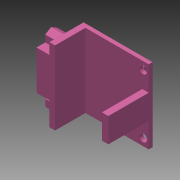
# Autodesk Inventor part: RS 232 Board
Saved by Autodesk Inventor 2015 SP1 (Build 190203100, 203)
## iProperties
Created: 2015-03-22
Part Number: RS 232 Board
Material: Generic
Document SubType Name: Modeling
Designer: steele
Density: 1 g/cm^3
Appearance: Pink
Author: steele
Autodesk Inventor part; units mm, degrees
ref_plane "YZ Plane" through (0, 0, 0) normal (1, 0, 0) x (0, 1, 0)
ref_plane "XZ Plane" through (0, 0, 0) normal (0, 1, 0) x (-1, 0, 0)
ref_plane "XY Plane" through (0, 0, 0) normal (0, 0, 1) x (1, 0, 0)
sketch "Sketch1" plane through (0, 0, 0) normal (0, 1, 0) x (-1, 0, 0)
  line L0 (14.5, -15.5) -> (-14.5, -15.5)
  line L1 (-14.5, -15.5) -> (-14.5, 15.5)
  line L2 (-14.5, 15.5) -> (14.5, 15.5)
  line L3 (14.5, 15.5) -> (14.5, -15.5)
  line L4 (14.5, -15.5) -> (-14.5, 15.5) construction
  line L5 (-14.5, -15.5) -> (14.5, 15.5) construction
  point P0 (0, 0)
  dimension "d0" = 29
  dimension "d1" = 31
  constraints: 12 end point, 2 midpoint, 2 parallel, 1 horizontal, 1 perpendicular
  measures "d0" distance of L0.start L0.end
  measures "d1" distance of L0.end L1.end
extrude "Extrusion1" add sketch "Sketch1" along normal blind 1.6
sketch "Sketch2" plane through (0, 0, 0) normal (0, -1, 0) x (1, 0, 0)
  line L0 (-14.5, 15.5) -> (-12.1, 15.5)
  line L1 (-12.1, 15.5) -> (-12.1, -15.5)
  line L2 (-12.1, -15.5) -> (-14.5, -15.5)
  line L3 (-14.5, -15.5) -> (-14.5, 15.5)
  point P0 (0, 0)
  dimension "d4" = 2.4
  constraints: 8 end point, 2 parallel, 1 horizontal, 1 perpendicular
  measures "d4" distance between parallel lines of L3 L1
extrude "Extrusion2" add sketch "Sketch2" along normal blind 12.8
sketch "Sketch3" plane through (0, 0, 0) normal (0, -1, 0) x (1, 0, 0)
  line L0 (-14.5, 15.5) -> (14.5, 15.5) construction
  line L1 (12.125, 15.5) -> (12.125, -15.5904) construction
  line L2 (14.5, -15.5) -> (14.5, 15.5) construction
  line L3 (12.125, 12.375) -> (14.5, 12.375) construction
  line L4 (12.125, -12.375) -> (14.5, -12.375) construction
  line L5 (-12.1, -15.5) -> (14.5, -15.5) construction
  circle A0 centre (12.125, 12.375) radius 1.625
  circle A1 centre (12.125, -12.375) radius 1.625
  point P0 (0, 0)
  dimension "d7" = 2.375
  dimension "d8" = 3.125
  dimension "d9" = 3.125
  dimension "d10" = 3.25
  constraints: 6 end point, 5 point on line, 2 centre point, 2 coincident, 1 equal radius, 1 parallel, 1 perpendicular, 1 vertical
  measures "d7" distance between parallel lines of L1 L2
  measures "d8" distance between parallel lines of L0 L3
  measures "d9" distance between parallel lines of L5 L4
  measures "d10" diameter of A0
extrude "Extrusion3" cut sketch "Sketch3" against normal through all
sketch "Sketch4" plane through (-14.5, 1.6, -15.5) normal (-1, 0, 0) x (0, 0, 1)
  line L0 (30.9539, -7.65) -> (0, -7.65) construction
  line L1 (0, -14.4) -> (0, 0) construction
  line L2 (0, 0) -> (31, 0) construction
  line L3 (24.3332, -7.65) -> (25.7766, -5.15)
  line L4 (25.7766, -5.15) -> (28.6634, -5.15)
  line L5 (28.6634, -5.15) -> (30.1068, -7.65)
  line L6 (30.1068, -7.65) -> (28.6634, -10.15)
  line L7 (28.6634, -10.15) -> (25.7766, -10.15)
  line L8 (25.7766, -10.15) -> (24.3332, -7.65)
  line L9 (2.3366, -10.15) -> (0.8932, -7.65)
  line L10 (0.8932, -7.65) -> (2.3366, -5.15)
  line L11 (2.3366, -5.15) -> (5.2234, -5.15)
  line L12 (5.2234, -5.15) -> (6.6668, -7.65)
  line L13 (6.6668, -7.65) -> (5.2234, -10.15)
  line L14 (5.2234, -10.15) -> (2.3366, -10.15)
  line L15 (31, 0) -> (31, -14.4) projected
  point P0 (15.5, -1.6)
  point P1 (27.22, -7.65)
  point P2 (3.78, -7.65)
  dimension "d13" = 7.65
  dimension "d14" = 5
  dimension "d15" = 3.78
  dimension "d16" = 3.78
  constraints: 26 end point, 3 parallel, 3 point on line, 1 horizontal, 26 other
  measures "d13" distance between parallel lines of L0 L2
  measures "d14" distance between parallel lines of L4 L7
  measures "d15" distance from line of L15 point (27.22, -7.65)
  measures "d16" distance from line of L1 point (3.78, -7.65)
extrude "Extrusion4" add sketch "Sketch4" along normal blind 6
sketch "Sketch5" plane through (-14.5, 1.6, -15.5) normal (-1, 0, 0) x (0, 0, 1)
  line L0 (0, 0) -> (31, 0) construction
  line L1 (15.5, 0) -> (15.5, -14.4) construction
  line L2 (31, -14.4) -> (0, -14.4) construction
  line L3 (23.75, -3.8) -> (7.25, -3.8)
  line L4 (7.25, -3.8) -> (7.25, -11.8)
  line L5 (7.25, -11.8) -> (23.75, -11.8)
  line L6 (23.75, -11.8) -> (23.75, -3.8)
  line L7 (23.75, -3.8) -> (7.25, -11.8) construction
  line L8 (7.25, -3.8) -> (23.75, -11.8) construction
  point P0 (15.5, -1.6)
  point P1 (15.5, -7.8)
  dimension "d19" = 3.8
  dimension "d20" = 8
  dimension "d21" = 16.5
  constraints: 14 end point, 4 midpoint, 2 parallel, 1 horizontal, 1 perpendicular, 1 point on line
  measures "d19" distance between parallel lines of L3 L0
  measures "d20" distance of L5.end L3.start
  measures "d21" distance of L4.end L5.end
extrude "Extrusion5" add sketch "Sketch5" along normal blind 8
sketch "Sketch6" plane through (0, 1.6, 0) normal (0, 1, 0) x (1, 0, 0)
  line L0 (9.5, -10.5) -> (9.5, 10.5)
  line L1 (9.5, 10.5) -> (-9.5, 10.5)
  line L2 (-9.5, 10.5) -> (-9.5, -10.5)
  line L3 (-9.5, -10.5) -> (9.5, -10.5)
  line L4 (9.5, -10.5) -> (-9.5, 10.5) construction
  line L5 (9.5, 10.5) -> (-9.5, -10.5) construction
  line L6 (14.5, -15.5) -> (14.5, 15.5) projected
  line L7 (-14.5, -15.5) -> (14.5, -15.5) projected
  point P0 (0, 0)
  dimension "d24" = 5
  dimension "d25" = 5
  constraints: 12 end point, 2 midpoint, 2 parallel, 1 perpendicular, 1 vertical
  measures "d24" distance between parallel lines of L0 L6
  measures "d25" distance between parallel lines of L3 L7
extrude "Extrusion6" add sketch "Sketch6" along normal blind 3
sketch "Sketch7" plane through (0, 0, 0) normal (0, -1, 0) x (1, 0, 0)
  line L0 (-12.1, 15.5) -> (-12.1, -15.5) construction
  line L1 (-12.1, 0) -> (14.5, 0) construction
  line L2 (14.5, 15.5) -> (14.5, -15.5) construction
  line L3 (14.5, -5.15) -> (14.5, 5.15)
  line L4 (14.5, 5.15) -> (11.8, 5.15)
  line L5 (11.8, 5.15) -> (11.8, -5.15)
  line L6 (11.8, -5.15) -> (14.5, -5.15)
  line L7 (14.5, -5.15) -> (11.8, 5.15) construction
  line L8 (14.5, 5.15) -> (11.8, -5.15) construction
  point P0 (0, 0)
  point P1 (13.15, 0)
  dimension "d28" = 10.3
  dimension "d29" = 2.7
  dimension "d30" = 0
  constraints: 14 end point, 4 midpoint, 2 parallel, 2 perpendicular, 1 point on line
  measures "d28" distance of L3.start L3.end
  measures "d29" distance of L3.end L4.end
  measures "d30" distance between parallel lines of L3 L2
extrude "Extrusion7" add sketch "Sketch7" along normal blind 17
body "Solid1"
